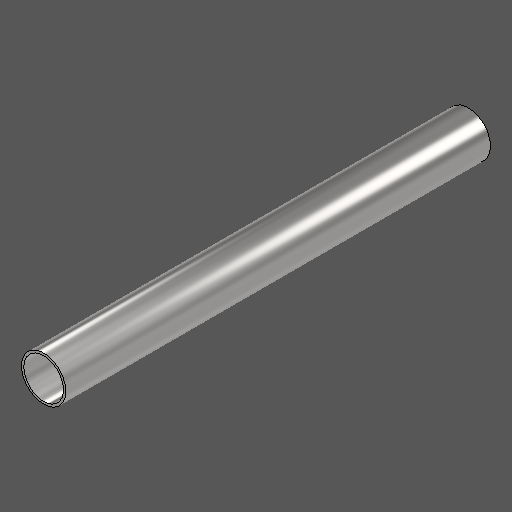
# Autodesk Inventor part: Electrode Skirt Pipe
Saved by Autodesk Inventor 2025 (Build 290162000, 162)
## iProperties
Created: 2024-05-17
Part Number: Electrode Skirt Pipe
Material: Stainless Steel
Document SubType Name: Modeling
Designer: KAA
Density: 8 g/cm^3
Appearance: Semi-Polished
Author: KAA
Autodesk Inventor part; units mm, degrees
ref_plane "YZ Plane" through (0, 0, 0) normal (1, 0, 0) x (0, 1, 0)
ref_plane "XZ Plane" through (0, 0, 0) normal (0, 1, 0) x (-1, 0, 0)
ref_plane "XY Plane" through (0, 0, 0) normal (0, 0, 1) x (1, 0, 0)
sketch "Sketch1" plane through (0, 0, 0) normal (0, 0, 1) x (1, 0, 0)
  circle A0 centre (0, 0) radius 5.15
  circle A1 centre (0, 0) radius 5.75
  dimension "d1" = 10.3
  dimension "d5" = 11.5
  constraints: 2 centre point, 2 coincident
  measures "d1" diameter of A0
  measures "d5" diameter of A1
extrude "Extrusion1" add sketch "Sketch1" along normal blind 110
body "Solid1"
